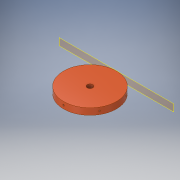
# Autodesk Inventor part: Avi Bay phenolic
Saved by Autodesk Inventor 2017 (Build 210142000, 142)
## iProperties
Created: 2016-11-08
Part Number: Avi Bay phenolic
Material: Phenolic Resin
Document SubType Name: Modeling
Designer: mnweir
Density: 1.38 g/cm^3
Appearance: Smooth - Light Orange
Author: mnweir
Autodesk Inventor part; units mm, degrees
ref_plane "YZ Plane" through (0, 0, 0) normal (1, 0, 0) x (0, 1, 0)
ref_plane "XZ Plane" through (0, 0, 0) normal (0, 1, 0) x (-1, 0, 0)
sketch "Sketch1" plane through (0, 0, 0) normal (0, 0, 1) x (1, 0, 0)
  line L0 (0, 0) -> (-88.9, 0)
  line L1 (-153.7877, 0) -> (0, 0)
  line L2 (-88.9, 0) -> (-88.9, -21.8948)
  line L3 (-88.9, -21.8948) -> (0, -21.8948)
  line L4 (0, -21.8948) -> (0, 0)
  dimension "d0" = 88.9
  dimension "d1" = 21.8948
  constraints: 10 end point, 2 horizontal, 1 perpendicular, 1 point on line, 1 vertical
  measures "d0" distance of L0.start L0.end
  measures "d1" distance of L0.end L2.end
revolve "Revolution1" add sketch "Sketch1" angle 360 about axis through (0, -21.8948, 0) along (0, 1, 0)
ref_plane "Work Plane1" through (0, -10.9474, -88.9) normal (0, 0, 1) x (1, 0, 0)
sketch "Sketch2" plane through (0, -10.9474, -88.9) normal (0, 0, 1) x (1, 0, 0)
  line L0 (0, 10.9474) -> (0, 0)
  dimension "d3" = 10.9474
  constraints: 2 end point, 1 vertical
  measures "d3" distance of L0.start L0.end
hole "Hole1" at (0, -10.9474, -88.9) direction (0, 0, 1) diameter 4.9784 depth 12.7 tip angle 118 thread size "1/4-20 UNC" class "2B" standard "ANSI Unified Screw Threads"
pattern_circular "Circular Pattern1" count 6 over 360 about axis through (0, -10, 0) along (0, 1, 0) of "Hole1"
sketch "Sketch3" plane through (0, 0, 0) normal (0, 1, 0) x (1, 0, 0)
  circle A0 centre (0, 0) radius 9.525
  point P0 (0, 0)
  dimension "d14" = 19.05
  constraints: 1 centre point, 1 coincident
  measures "d14" diameter of A0
extrude "Extrusion1" cut sketch "Sketch3" against normal blind 74.6125
body "Solid1"
